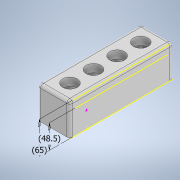
# Autodesk Inventor part: Full
Saved by Autodesk Inventor 2021 (Build 250183000, 183)
## iProperties
Created: 2020-05-12
Part Number: Full
Material: Generic
Document SubType Name: Modeling
Designer: andre
Density: 1 g/cm^3
Appearance: Default
Author: andre
Autodesk Inventor part; units mm, degrees
ref_plane "YZ Plane" through (0, 0, 0) normal (1, 0, 0) x (0, 1, 0)
ref_plane "XZ Plane" through (0, 0, 0) normal (0, 1, 0) x (-1, 0, 0)
ref_plane "XY Plane" through (0, 0, 0) normal (0, 0, 1) x (1, 0, 0)
sketch "Base" plane through (0, 0, 0) normal (0, 1, 0) x (-1, 0, 0)
  line L0 (0, 35) -> (0, -175)
  line L1 (0, -175) -> (65, -175)
  line L2 (65, -175) -> (65, 35)
  line L3 (65, 35) -> (0, 35)
  dimension "d6" = 210
  dimension "d7" = 65
  constraints: 8 end point, 2 perpendicular, 1 vertical
  measures "d6" distance between parallel lines of L1 L3
  measures "d7" distance of L0.end L1.end
extrude "Extrusion2" add sketch "Base" along normal blind 65
sketch "Top" plane through (0, 65, 0) normal (0, 1, 0) x (1, 0, 0)
  circle A0 centre (-32.5, 46) radius 17
  circle A1 centre (-32.5, -2) radius 17
  circle A2 centre (-32.5, 94) radius 17
  circle A3 centre (-32.5, 142) radius 17
  line L0 (0, 175) -> (-65, 175) projected
  line L1 (-65, 175) -> (-65, -35) projected
  line L2 (-65, -35) -> (0, -35) construction
  line L3 (-32.5, -35) -> (-32.5, 175) construction
  circle A4 centre (-32.5, -2) radius 15
  circle A5 centre (-32.5, 46) radius 15
  circle A6 centre (-32.5, 94) radius 15
  circle A7 centre (-32.5, 142) radius 15
  point P0 (-32.5, 70)
  dimension "d10" = 34
  dimension "d11" = 34
  dimension "d12" = 34
  dimension "d13" = 34
  dimension "d14" = 48
  dimension "d15" = 48
  dimension "d16" = 48
  dimension "d27" = 30
  dimension "d28" = 30
  dimension "d29" = 30
  dimension "d30" = 30
  dimension "d31" = 24
  dimension "d32" = 105
  dimension "d35" = 33
  constraints: 8 centre point, 4 coincident, 3 midpoint, 3 vertical alignment, 2 end point, 1 point on line
  measures "d10" diameter of A0
  measures "d11" diameter of A1
  measures "d12" diameter of A2
  measures "d13" diameter of A3
  measures "d14" distance of A0.centre A1.centre
  measures "d15" distance of A2.centre A0.centre
  measures "d16" distance of A3.centre A2.centre
  measures "d27" diameter of A4
  measures "d28" diameter of A5
  measures "d29" diameter of A6
  measures "d30" diameter of A7
  measures "d31" distance of point (-32.5, 70) A2.centre
  measures "d32" distance from line of point (-32.5, 70) L0
  measures "d35" distance from line of A1.centre L2
extrude "Extrusion3" cut sketch "Top" against normal up to next contours A4 | A5 | A6 | A7
sketch "Walls" plane through (0, 0, 0) normal (0, -1, 0) x (1, 0, 0)
  line L0 (-11, 24) -> (-54, 24)
  line L1 (-54, 24) -> (-54, -164)
  line L2 (-54, -164) -> (-11, -164)
  line L3 (-11, -164) -> (-11, 24)
  line L4 (-65, 35) -> (0, 35) projected
  line L5 (0, -175) -> (-65, -175) projected
  line L6 (0, 35) -> (0, -175) projected
  line L7 (-65, -175) -> (-65, 35) projected
  point P0 (0, 0)
  dimension "d21" = 11
  dimension "d22" = 11
  dimension "d23" = 11
  dimension "d24" = 11
  dimension "d33" = 43
  constraints: 8 end point, 2 parallel, 1 horizontal, 1 perpendicular
  measures "d21" distance between parallel lines of L4 L0
  measures "d22" distance between parallel lines of L5 L2
  measures "d23" distance between parallel lines of L6 L3
  measures "d24" distance between parallel lines of L7 L1
  measures "d33" distance between parallel lines of L1 L3
extrude "Extrusion4" cut sketch "Walls" against normal blind 48.5 contours L3 L2 L1 L0
sketch "Sketch6" plane through (0, 0, 35) normal (1, 0, 0) x (0, 0, -1)
  line L0 (0, 0) -> (210, 0) projected
  line L1 (11, 48.5) -> (199, 48.5) projected
  point P0 (35, 0)
  point P1 (33.3852, 33.5)
  dimension "d34" = 48.5
  constraints: 1 other
fillet "Fillet1" radius 6 8 edges at (-32.5, 65, 35) (-65, 65, -70) (0, 65, -70) (0, 32.5, 35) (-65, 32.5, 35) (0, 32.5, -175) (-32.5, 65, -175) (-65, 32.5, -175)
sketch "Sketch7" plane through (-65, 0, -169) normal (-1, 0, 0) x (0, 0, 1)
  line L0 (0, 59) -> (198, 59) projected
  line L1 (99, 59) -> (99, 0) construction
  line L2 (0, 0) -> (198, 0) projected
  circle A0 centre (99, 0) radius 6.35
  point P0 (169, 0)
  dimension "d40" = 12.7
  constraints: 2 end point, 2 midpoint, 1 centre point
  measures "d40" diameter of A0
extrude "Extrusion5" cut sketch "Sketch7" against normal up to surface (11 mm away)
fillet "Fillet2" radius 6 4 edges at (-11, 24.25, 24) (-54, 24.25, 24) (-11, 24.25, -164) (-54, 24.25, -164)
sketch "Sketch8" plane through (0, 0, 29) normal (1, 0, 0) x (0, 0, -1)
  line L0 (0, 0) -> (198, 0) projected
  line L1 (198, 65) -> (0, 65) projected
  point P0 (29, 0)
  dimension "d42" = 65
  measures "d42" distance between parallel lines of L0 L1
fillet "Fillet3" radius 1.5 8 edges at (-52.2426, 48.5, 22.2426) (-32.5, 48.5, 24) (-12.7574, 48.5, 22.2426) (-11, 48.5, -70) (-12.7574, 48.5, -162.2426) (-32.5, 48.5, -164) (-52.2426, 48.5, -162.2426) (-54, 48.5, -70)
equation "\"d8\" = d7"
equation "\"d11\" = d10"
equation "\"d12\" = d10"
equation "\"d13\" = d10"
equation "\"d15\" = d14"
equation "\"d16\" = d14"
equation "\"d28\" = d27"
equation "\"d29\" = d27"
equation "\"d30\" = d27"
equation "\"d31\" = 0.5 * d14"
equation "\"d32\" = 0.5 * d6"
equation "\"d22\" = d21"
equation "\"d23\" = d21"
equation "\"d24\" = d23"
equation "\"d25\" = d7 - 1.5 * d21"
equation "\"d41\" = d36"
equation "\"d43\" = 0.25 * d36"
equation "\"d36\" = 6"
body "Solid2"
